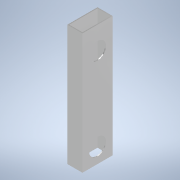
# Autodesk Inventor part: 2x1 Front
Saved by Autodesk Inventor 2020 (Build 240168000, 168)
## iProperties
Created: 2020-01-27
Part Number: 2x1 Front
Material: Aluminum 6061
Document SubType Name: Modeling
Designer: 1cikaychapman
Density: 2.7 g/cm^3
Appearance: Aluminum - Flat
Author: 1cikaychapman
Autodesk Inventor part; units mm, degrees
ref_plane "YZ Plane" through (0, 0, 0) normal (1, 0, 0) x (0, 1, 0)
ref_plane "XZ Plane" through (0, 0, 0) normal (0, 1, 0) x (-1, 0, 0)
ref_plane "XY Plane" through (0, 0, 0) normal (0, 0, 1) x (1, 0, 0)
sketch "Sketch1" plane through (0, 0, 0) normal (0, 1, 0) x (-1, 0, 0)
  line L0 (-12.7, 25.4) -> (12.7, 25.4)
  line L1 (12.7, 25.4) -> (12.7, -25.4)
  line L2 (12.7, -25.4) -> (-12.7, -25.4)
  line L3 (-12.7, -25.4) -> (-12.7, 25.4)
  line L4 (-12.7, 25.4) -> (12.7, -25.4) construction
  line L5 (12.7, 25.4) -> (-12.7, -25.4) construction
  line L6 (11.1125, 23.8125) -> (-11.1125, 23.8125)
  line L7 (-11.1125, 23.8125) -> (-11.1125, -23.8125)
  line L8 (-11.1125, -23.8125) -> (11.1125, -23.8125)
  line L9 (11.1125, -23.8125) -> (11.1125, 23.8125)
  line L10 (11.1125, 23.8125) -> (-11.1125, -23.8125) construction
  line L11 (-11.1125, 23.8125) -> (11.1125, -23.8125) construction
  point P0 (0, 0)
  dimension "d0" = 25.4
  dimension "d1" = 50.8
  dimension "d2" = 22.225
  dimension "d3" = 47.625
  constraints: 24 end point, 4 midpoint, 4 parallel, 2 horizontal, 2 perpendicular
  measures "d0" distance of L1.end L2.end
  measures "d1" distance of L0.end L1.end
  measures "d2" distance of L8.end L7.end
  measures "d3" distance of L7.end L6.end
extrude "Extrusion1" add sketch "Sketch1" along normal blind 203.2
sketch "Sketch2" plane through (12.7, 0, 25.4) normal (1, 0, 0) x (0, 0, -1)
  line L0 (0, 203.2) -> (50.8, 203.2) projected
  line L1 (0, 0) -> (0, 203.2) projected
  point P0 (25.4, 0)
  point P1 (25.4, 165.1)
  dimension "d20" = 38.1
  dimension "d21" = 25.4
  measures "d20" distance from line of L0 point (25.4, 165.1)
  measures "d21" distance from line of L1 point (25.4, 165.1)
hole "Hole1" at (12.7, 165.1, 0) direction (-1, 0, 0) diameter 28.575 end through all
sketch "Sketch3" plane through (12.7, 0, 25.4) normal (1, 0, 0) x (0, 0, -1)
  line L0 (50.8, 0) -> (50.8, 203.2) projected
  line L1 (0, 0) -> (50.8, 0) projected
  point P0 (25.4, 0)
  point P1 (25.4, 25.4)
  dimension "d22" = 25.4
  dimension "d23" = 25.4
  measures "d22" distance from line of L0 point (25.4, 25.4)
  measures "d23" distance from line of L1 point (25.4, 25.4)
hole "Hole2" at (12.7, 25.4, 0) direction (-1, 0, 0) diameter 28.575 end through all
body "Solid1"
